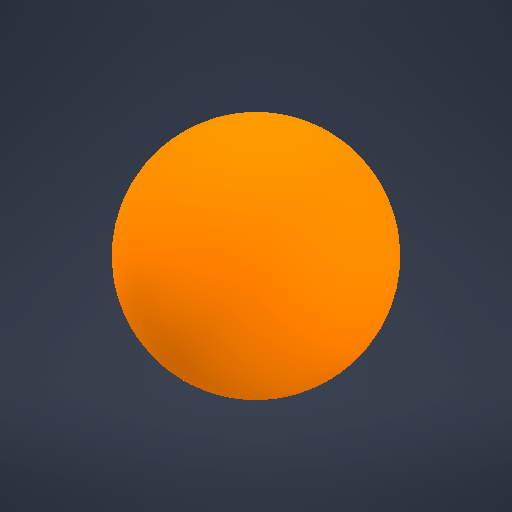
# Autodesk Inventor part: TT_BALL
Saved by Autodesk Inventor 2027.1 (Build 311270010, 270A)
## iProperties
Created: 2026-08-27
Part Number: TT_BALL
Material: Generic
Document SubType Name: Modeling
Designer: RIDDHIMAN
Density: 1 g/cm^3
Appearance: Default
Author: RIDDHIMAN
Autodesk Inventor part; units mm, degrees
ref_plane "YZ Plane" through (0, 0, 0) normal (1, 0, 0) x (0, 1, 0)
ref_plane "XZ Plane" through (0, 0, 0) normal (0, 1, 0) x (-1, 0, 0)
ref_plane "XY Plane" through (0, 0, 0) normal (0, 0, 1) x (1, 0, 0)
sketch "Sketch1" plane through (0, 0, 0) normal (0, 0, 1) x (1, 0, 0)
  arc A0 (20, 0) -> (-20, 0) centre (0, 0) ccw
  arc A1 (19.5, 0) -> (-19.5, 0) centre (0, 0) ccw
  line L0 (-20, 0) -> (-19.5, 0)
  line L1 (19.5, 0) -> (20, 0)
  line L2 (-28, 0) -> (28, 0) projected
  constraints: 4 end point, 4 point on circle, 2 centre point, 2 coincident, 2 horizontal
revolve "Revolution1" add sketch "Sketch1" angle 360 about axis through (-10, 0, 0) along (1, 0, 0) contours L1 A1 L0 A0
body "Solid1"
